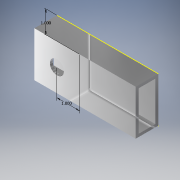
# Autodesk Inventor part: 15102898-16-P-0304
Saved by Autodesk Inventor 2017 (Build 210142000, 142)
## iProperties
Created: 2016-10-03
Part Number: 15102898-16-P-0304
Material: Aluminum 6061
Document SubType Name: Modeling
Designer: gus
Density: 2.7 g/cm^3
Appearance: Aluminum - Flat
Author: gus
Autodesk Inventor part; units mm, degrees
ref_plane "YZ Plane" through (0, 0, 0) normal (1, 0, 0) x (0, 1, 0)
ref_plane "XZ Plane" through (0, 0, 0) normal (0, 1, 0) x (-1, 0, 0)
ref_plane "XY Plane" through (0, 0, 0) normal (0, 0, 1) x (1, 0, 0)
sketch "Sketch1" plane through (0, 0, 0) normal (1, 0, 0) x (0, 1, 0)
  line L0 (0, 0) -> (50.8, 0)
  line L1 (50.8, 0) -> (50.8, -25.4)
  line L2 (50.8, -25.4) -> (0, -25.4)
  line L3 (0, -25.4) -> (0, 0)
  line L4 (47.625, -3.175) -> (3.175, -3.175)
  line L5 (3.175, -3.175) -> (3.175, -22.225)
  line L6 (3.175, -22.225) -> (47.625, -22.225)
  line L7 (47.625, -22.225) -> (47.625, -3.175)
  dimension "d0" = 50.8
  dimension "d1" = 25.4
  dimension "d2" = 3.175
  constraints: 16 end point, 4 parallel, 2 perpendicular, 1 horizontal, 3 other
  measures "d0" distance of L1.end L2.end
  measures "d1" distance of L0.end L1.end
  measures "d2" distance between parallel lines of L0 L4
extrude "Extrusion1" add sketch "Sketch1" along normal blind 114.3
sketch "Sketch2" plane through (0, 0, -25.4) normal (0, 0, -1) x (-1, 0, 0)
  line L0 (0, 50.8) -> (-114.3, 50.8) projected
  line L1 (0, 50.8) -> (0, 0) projected
  line L2 (0, 0) -> (-114.3, 0) projected
  point P0 (-25.4, 25.4)
  dimension "d5" = 25.4
  dimension "d6" = 25.4
  measures "d5" distance from line of L0 point (-25.4, 25.4)
  measures "d6" distance from line of L1 point (-25.4, 25.4)
hole "Hole1" at (25.4, 25.4, -25.4) direction (0, 0, 1) diameter 28.575 depth 3.175 tip angle 118
hole "Hole2" at (25.4, 25.4, -25.4) direction (0, 0, 1) diameter 15.875 end through all
body "Solid1"
